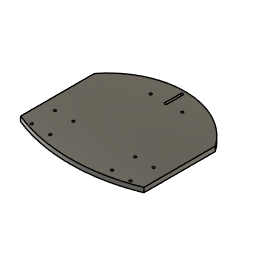
自制车架 (Autodesk Fusion 360 design; units mm, degrees)
Autodesk Fusion 360 part; units mm, degrees
note: some values were not read from the file. Set by a fixed rule: which sketch regions a step uses.
sketch "草图1" plane through (0, 0, 0) normal (0, 0, 1) x (1, 0, 0)
  line L0 (-80, -84.3478) -> (-80, 11.2707)
  line L1 (80, -84.3478) -> (80, 8.2588)
  circle A0 centre (-64, -85.6725) radius 1.5
  circle A1 centre (-40, -85.6725) radius 1.5
  circle A2 centre (-64, -55.6725) radius 1.5
  circle A3 centre (-40, -55.6725) radius 1.5
  circle A4 centre (40, -55.6725) radius 1.5
  circle A5 centre (64, -55.6725) radius 1.5
  circle A6 centre (40, -85.6725) radius 1.5
  circle A7 centre (64, -85.6725) radius 1.5
  circle A8 centre (-20.5, 25) radius 1.5
  circle A9 centre (20.5, 25) radius 1.5
  line L2 (-1.5, 45) -> (-1.5, 24)
  arc A10 (-1.5, 24) -> (1.5, 24) centre (0, 24) ccw
  line L3 (1.5, 24) -> (1.5, 45)
  arc A11 (1.5, 45) -> (-1.5, 45) centre (0, 45) ccw
  line L4 (0, 46.5) -> (0, 22.5) construction
  arc A12 (80, 8.2588) -> (-80, 11.2707) centre (-1.119, -49.6781) ccw
  arc A13 (-80, -84.3478) -> (80, -84.3478) centre (0, 112.2701) ccw
  point P0 (0, 50)
  dimension "d4" = 3
  dimension "d7" = 24
  dimension "d8" = 30
  dimension "d9" = 40
  dimension "d10" = 3
  dimension "d11" = 30
  dimension "d14" = 24
  dimension "d15" = -30
  dimension "d16" = 40
  dimension "d17" = 3
  dimension "d22" = 20.5
  dimension "d24" = 20.5
  dimension "d25" = 41
  dimension "d26" = 3
  dimension "d29" = 80
  dimension "d30" = 80
  dimension "d33" = 5
  constraint tangent L2 A10
  constraint tangent A10 L3
  constraint parallel L2 L3
  constraint tangent L3 A11
  constraint tangent L2 A11
  constraint midpoint A11 L4.start
  constraint midpoint A10 L4.end
  constraint vertical L4
  constraint vertical L0
  constraint vertical L1
  constraint coincident A12 P0
  measures "d4" diameter of A0
  measures "d9" horizontal distance of origin A3.centre
  measures "d10" diameter of A4
  measures "d11" vertical distance of A1.centre A4.centre
  measures "d16" horizontal distance of origin A4.centre
  measures "d17" diameter of A8
  measures "d22" horizontal distance of origin A8.centre
  measures "d24" horizontal distance of origin A9.centre
  measures "d25" distance of A8.centre A9.centre
  measures "d26" diameter of A10
  measures "d29" distance of origin L0
  measures "d30" distance of origin L1
  measures "d33" distance of A11.centre P0
extrude "拉伸1" add sketch "草图1" along normal blind 2
extrude "拉伸2" add sketch "草图1" along normal blind 6
equation "d22 = 19 mm + 1.5 mm"
equation "d25 = 38 mm + 3 mm"
